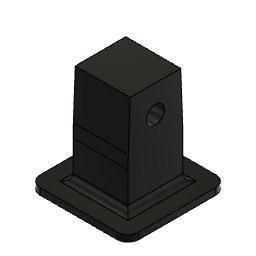
Wall pad (Autodesk Fusion 360 design; units mm, degrees)
Autodesk Fusion 360 part; units mm, degrees
box "BoitePrimitive1" add length 25 width 25 height 25 placed x (0, 0, 1) y (1, 0, 0) z (0, 1, 0) at (0, 0, 0)
hole "Perçage1" at (25, 12.5, 12.5) direction (-1, 0, 0) diameter 8.2 end through all
move_face "DécalerLesFaces1" offset 20 1 faces at (16.6667, 0, 8.3333)
sketch "Esquisse4" plane through (0, -20, 0) normal (0, -1, 0) x (1, 0, 0)
  line L0 (25, 25) -> (0, 25)
  line L1 (0, 25) -> (0, 0)
  line L2 (0, 0) -> (25, 0)
  line L3 (25, 0) -> (25, 25)
  line L4 (-10, -10) -> (35, -10)
  line L5 (35, -10) -> (35, 35)
  line L6 (35, 35) -> (-10, 35)
  line L7 (-10, 35) -> (-10, -10)
  dimension "d13" = 10
extrude "Extrusion1" add sketch "Esquisse4" along normal blind 3 contours L0 L1 L2 L3 | L4 L5 L6 L7
chamfer "Chanfrein1" distance 1 distance2 25 2 edges at (12.5, 25, 25) (12.5, 25, 0) measured on face at (16.6667, 25, 8.3333) measured on face at (16.6667, 25, 8.3333)
fillet "Congé2" radius 150 2 edges at (12.5, 0, 25) (12.5, 0, 0)
fillet "Congé1" radius 5 4 edges at (35, -21.5, 35) (-10, -21.5, 35) (35, -21.5, -10) (-10, -21.5, -10)
fillet "Congé3" radius 3 4 edges at (12.5, -20, 25) (25, -20, 12.5) (12.5, -20, 0) (0, -20, 12.5)
equation "base_l = 25 mm"
equation "d2 = base_l"
equation "d3 = base_l"
equation "d4 = base_l"
equation "d8 = trou_diam + trou_delta"
equation "trou_diam = 8 mm"
equation "trou_delta = 0.2 mm"
equation "d12 = base_l - 5 mm"
equation "d13 = empattement"
equation "d14 = ep"
equation "ep = 3 mm"
equation "empattement = 10 mm"
equation "d19 = base_l / 5"
equation "d21 = base_l"
named bodies: "Wall pad"
